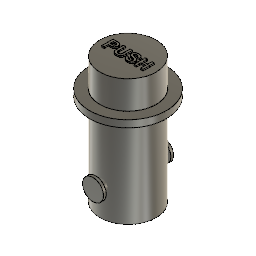
push button v5 (Autodesk Fusion 360 design; units mm, degrees)
Autodesk Fusion 360 part; units mm, degrees
sketch "Sketch1" plane through (0, 0, 0) normal (0, 0, 1) x (1, 0, 0)
  circle A0 centre (0, 0) radius 20
  dimension "d1" = 40
  constraint coincident A0.centre origin
  measures "d1" diameter of A0
extrude "Extrude1" add sketch "Sketch1" along normal blind 90 makes body 1
sketch "Sketch2" plane through (0, 0, 0) normal (0, 1, 0) x (1, 0, 0)
  circle A0 centre (0, -20) radius 5
  line L0 (-20, -90) -> (20, -90)
  line L1 (-20, 0) -> (20, 0)
  dimension "d4" = 10
  dimension "d24" = 20
  measures "d4" diameter of A0
  measures "d24" distance of A0.centre L1
extrude "Extrude2" add sketch "Sketch2" along normal mid plane 50 separate body makes body 2
sketch "Sketch3" plane through (0, 0, 90) normal (0, 0, 1) x (-1, 0, 0)
  circle A0 centre (0, 0) radius 20
  circle A1 centre (0, 0) radius 20
  line L0 (20, -20) -> (-20, -20)
  line L1 (-20, -20) -> (-20, 20)
  line L2 (-20, 20) -> (20, 20)
  line L3 (20, 20) -> (20, -20)
  line L4 (20, 20) -> (-20, 20) construction
  line L5 (-20, 20) -> (-20, -20) construction
  line L6 (-20, -20) -> (20, -20) construction
  line L7 (20, -20) -> (20, 20) construction
  dimension "d10" = 40
  dimension "d11" = 40
  dimension "d12" = 40
  dimension "d13" = 8
  text T0 "PUSH" font "Arial" height 8 bold align centre middle in box 40 x 40 at (20, 20) x (-1, 0) y (0, -1) spacing 1
  constraint coincident A0.centre A1.centre
  constraint horizontal L0
  constraint vertical L1
  constraint horizontal L2
  constraint vertical L3
  constraint tangent A1 L1
  constraint tangent A1 L0
  constraint coincident L1.end
  constraint coincident L0.start
  measures "d10" diameter of A1
  measures "d11" distance of L0.start L0.end
  measures "d12" distance of L0.start L2.end
extrude "Extrude3" add sketch "Sketch3" along normal blind 1 text T0 bodies 1
sketch "Sketch4" plane through (0, -25, 0) normal (0, -1, 0) x (1, 0, 0)
  circle A0 centre (0, 20) radius 5
  circle A1 centre (0, 20) radius 7.5
  dimension "d16" = 15
  constraint concentric A0 A1
  measures "d16" diameter of A1
extrude "Extrude4" add sketch "Sketch4" against normal blind 2 bodies 2
sketch "Sketch5" plane through (0, 25, 0) normal (0, 1, 0) x (-1, 0, 0)
  circle A0 centre (0, 20) radius 5
  circle A1 centre (0, 20) radius 7.5
  dimension "d19" = 15
  constraint concentric A0 A1
  measures "d19" diameter of A1
extrude "Extrude5" add sketch "Sketch5" against normal blind 2 bodies 2
ref_plane "WorkPlane1" through (0, 0, 80) normal (0, 0, 1) x (1, 0, 0)
sketch "Sketch6" plane through (0, 0, 80) normal (0, 0, 1) x (1, 0, 0)
  circle A0 centre (0, 0) radius 27.5
  dimension "d23" = 55
  constraint coincident A0.centre origin
  measures "d23" diameter of A0
extrude "Extrude6" add sketch "Sketch6" against normal blind 15 bodies 1
extrude "Extrude7" cut 1 faces at (24.8232, -2.3598, 80) along direction (0, 0, -1) blind 10 on bodies 1 bodies 1
